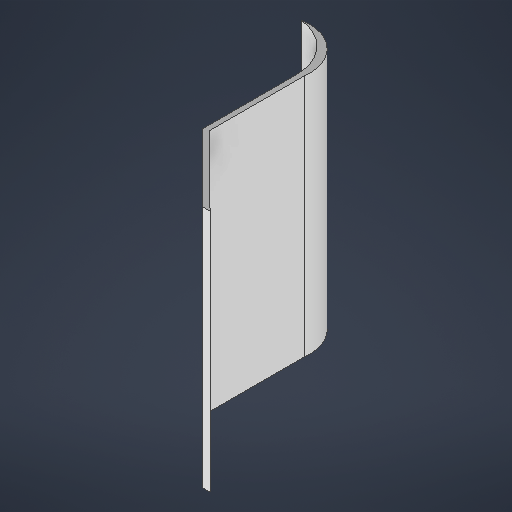
# Autodesk Inventor part: tampa mini sumôipt
Saved by Autodesk Inventor 2026.1 (Build 301233000, 233)
## iProperties
Created: 2025-11-14
Part Number: tampa mini sumôipt
Material: Genérico
Document SubType Name: Modeling
Designer: panto
Density: 1 g/cm^3
Appearance: Padrão
Author: panto
Autodesk Inventor part; units mm, degrees
ref_plane "YZ Plane" through (0, 0, 0) normal (1, 0, 0) x (0, 1, 0)
ref_plane "XZ Plane" through (0, 0, 0) normal (0, 1, 0) x (-1, 0, 0)
ref_plane "XY Plane" through (0, 0, 0) normal (0, 0, 1) x (1, 0, 0)
sketch "Esboço1" plane through (0, 0, 0) normal (0, 1, 0) x (-1, 0, 0)
  line L0 (-15.6873, 39.0494) -> (11.3127, 12.0494)
  line L1 (-16.1105, 36.3428) -> (9.2885, 10.9439)
  line L2 (9.2885, 10.9439) -> (9.2885, -27.0561)
  line L3 (11.3127, 12.0494) -> (11.3127, -25.9506)
  line L4 (29.3127, -45.9506) -> (29.3127, -45.8503)
  arc A0 (9.2885, -27.0561) -> (29.3127, -45.8503) centre (26.1596, -29.1453) ccw
  line L5 (-16.1105, 36.3428) -> (-18.8894, 39.0494)
  line L6 (-18.8894, 39.0494) -> (-15.6873, 39.0494)
  line L7 (-18.8894, 39.0494) -> (-15.6873, 39.0494)
  line L8 (-15.6873, 39.0494) -> (11.3127, 12.0494)
  line L9 (11.3127, 12.0494) -> (11.3127, -25.9506)
  arc A1 (11.3127, -25.9506) -> (29.3127, -45.8503) centre (31.3127, -25.9506) ccw
  arc A2 (11.3127, -25.9506) -> (29.3127, -45.8503) centre (31.3127, -25.9506) ccw
  point P0 (0, 0)
  dimension "d0" = 17
  constraints: 20 end point, 6 point on circle, 3 centre point, 2 parallel, 1 collinear
  measures "d0" radius of A0
extrude "Extrusão1" add sketch "Esboço1" along normal blind 98
